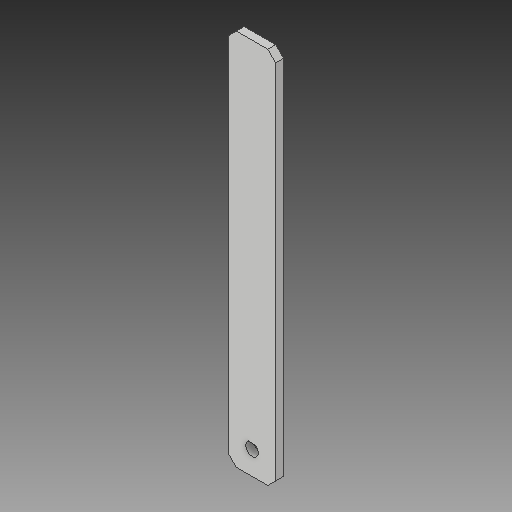
# Autodesk Inventor part: arm_distal
Saved by Autodesk Inventor 2019 (Build 230136000, 136)
## iProperties
Created: 2019-05-15
Part Number: arm_distal
Material: Generic
Document SubType Name: Modeling
Designer: Nathan
Density: 1 g/cm^3
Appearance: Default
Author: Nathan
Autodesk Inventor part; units mm, degrees
ref_plane "YZ Plane" through (0, 0, 0) normal (1, 0, 0) x (0, 1, 0)
ref_plane "XZ Plane" through (0, 0, 0) normal (0, 1, 0) x (-1, 0, 0)
ref_plane "XY Plane" through (0, 0, 0) normal (0, 0, 1) x (1, 0, 0)
sketch "Sketch1" plane through (0, 0, 0) normal (0, 0, 1) x (1, 0, 0)
  line L0 (-9.525, 0) -> (9.525, 0)
  line L1 (9.525, 0) -> (9.525, 152.4)
  line L2 (9.525, 152.4) -> (-9.525, 152.4)
  line L3 (-9.525, 152.4) -> (-9.525, 0)
  point P0 (0, 0)
  point P1 (0, 0)
  dimension "d0" = 19.05
  dimension "d1" = 152.4
  constraints: 8 end point, 2 parallel, 1 coincident, 1 horizontal, 1 horizontal alignment, 1 midpoint, 1 perpendicular
  measures "d0" distance of L2.end L1.end
  measures "d1" distance of L1.end L0.end
extrude "Extrusion1" add sketch "Sketch1" along normal blind 3.175
sketch "Sketch2" plane through (0, 0, 3.175) normal (0, 0, 1) x (1, 0, 0)
  arc A0 (-1.5, 11.5881) -> (1.5, 11.5881) centre (0, 9.525) ccw
  line L0 (-1.5, 11.5881) -> (1.5, 11.5881)
  line L1 (9.525, 0) -> (9.525, 152.4) projected
  line L2 (-9.525, 0) -> (9.525, 0) projected
  point P0 (0, 0)
  point P1 (0, 0)
  dimension "d4" = 2.5508
  dimension "d5" = 3
  dimension "d8" = 9.525
  dimension "d9" = 9.525
  constraints: 2 end point, 2 point on circle, 1 centre point, 1 horizontal, 1 midpoint, 1 vertical alignment
  measures "d4" radius of A0
  measures "d5" distance of L0.start L0.end
  measures "d8" distance from line of L1 A0.centre
  measures "d9" distance of point (0, 0) A0.centre
extrude "Extrusion2" cut sketch "Sketch2" against normal blind 3.175
chamfer "Chamfer1" distance 3.175 angle 45 4 edges at (9.525, 0, 1.5875) (-9.525, 0, 1.5875) (9.525, 152.4, 1.5875) (-9.525, 152.4, 1.5875)
equation "\"d0\" = arm_distal_width"
equation "\"d1\" = arm_distal_length"
equation "\"d2\" = arm_distal_thickness"
equation "\"d9\" = d8"
equation "\"d10\" = arm_distal_thickness"
equation "\"base_width\" = 127"
equation "\"base_length\" = 177.8"
equation "\"base_height\" = 12.7"
equation "\"base_motor_standoff_length\" = 63.5"
equation "\"base_motor_standoff_height\" = 12.7"
equation "\"base_motor_standoff_thickness\" = 3.175"
equation "\"base_motor_standoff_offset\" = 0"
equation "\"waist_motor_cutout_diameter\" = 50.8"
equation "\"waist_cutout_overlap\" = 6.35"
equation "\"retention_poles_diameter\" = 6.35"
equation "\"turntable_bed_depth\" = 0"
equation "\"turntable_diameter\" = 101.6"
equation "\"turntable_spur_thickness\" = 6.35"
equation "\"turntable_thickness\" = 9.525"
equation "\"spine_diameter\" = 31.75"
equation "\"shoulder_height_offset\" = 25.4"
equation "\"shoulder_width\" = 69.85"
equation "\"shoulder_length\" = 50.8"
equation "\"shoulder_wall_thickness\" = 4.7625"
equation "\"arm_proximal_gear_diameter\" = 63.5"
equation "\"arm_proximal_gear_thickness\" = 9.525"
equation "\"shoulder_motor_gear_diameter\" = 25.4"
equation "\"arm_proximal_length\" = 203.2"
equation "\"arm_proximal_width\" = 12.7"
equation "\"arm_distal_length\" = 152.4"
equation "\"arm_distal_width\" = 19.05"
equation "\"arm_distal_thickness\" = 3.175"
equation "\"arm_proximal_thickness\" = 9.525"
equation "\"shoulder_motor_boss\" = 25.4"
equation "\"shoulder_gear_shaft_diameter\" = 12.7"
equation "\"shoulder_gear_thickness\" = 6.35"
equation "\"shoulder_gear_diameter\" = 63.5"
equation "\"spine_height\" = 25.4"
equation "\"turntable_retention_shaft_length\" = 152.4"
equation "\"turntable_height\" = 9.525"
equation "\"turntable_spur_width\" = 6.35"
equation "\"turntable_retention_shaft_diameter\" = 6.35"
equation "\"turntable_motor_support_width\" = 63.5"
equation "\"turntable_motor_boss\" = 25.4"
equation "\"turntable_motor_support_height\" = 25.4"
equation "\"turntable_motor_support_thickness\" = 3.175"
equation "\"base_cutout_diameter\" = 44.45"
equation "\"base_cutout_contact_angle\" = 70deg"
equation "\"arm_proximal_central_diameter\" = 25.4"
equation "\"arm_proximal_motor_boss\" = 25.4"
equation "\"turntable_ring_height\" = 9.525"
equation "\"turntable_ring_diameter\" = 19.05"
body "Solid1"
